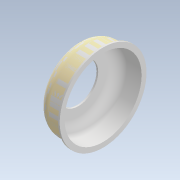
# Autodesk Inventor part: cazoleta
Saved by Autodesk Inventor 2021 (Build 250183000, 183)
## iProperties
Created: 2021-04-24
Part Number: cazoleta
Material: Genérico
Document SubType Name: Modeling
Designer: j2seb
Density: 1 g/cm^3
Appearance: Valor por defecto
Author: j2seb
Autodesk Inventor part; units mm, degrees
ref_plane "YZ Plane" through (0, 0, 0) normal (1, 0, 0) x (0, 1, 0)
ref_plane "XZ Plane" through (0, 0, 0) normal (0, 1, 0) x (-1, 0, 0)
ref_plane "XY Plane" through (0, 0, 0) normal (0, 0, 1) x (1, 0, 0)
sketch "Boceto1" plane through (0, 0, 0) normal (0, 0, 1) x (1, 0, 0)
  line L0 (0, 12) -> (0, 17.5)
  arc A0 (7, 24.5) -> (0, 17.5) centre (7, 17.5) ccw
  line L1 (7, 24.5) -> (15, 24.5)
  line L2 (15, 24.5) -> (15, 26.5)
  line L3 (0, 0) -> (11, 0)
  dimension "d0" = 49
  dimension "d1" = 15
  dimension "d2" = 2
  dimension "d3" = 7
  dimension "d4" = 12
  constraints: 8 end point, 2 horizontal, 2 point on circle, 2 tangent, 1 centre point, 1 perpendicular, 1 point on line, 1 vertical
  measures "d0" diameter of L1 L3
  measures "d1" distance from line of L3.start L2
  measures "d2" distance of L1.end L2.end
  measures "d3" radius of A0
  measures "d4" distance of L3.start L0.start
surface revolve "SuperficieRevolución1" sketch "Boceto1" angle 360 about axis through (0, 0, 0) along (1, 0, 0) shown yes curves L2 L1 A0 L0
thicken "Engrosado1" operation new thickness 1 both sides no extend neighbours no toward (1, 0, 0) faces at (15, 25.5767, -2.114) (12.3333, 24.4206, -1.9714) (6.4769, 24.1634, -3.9269) (0, 15.4972, -1.396)
